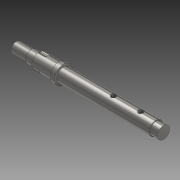
# Autodesk Inventor part: thumb_03 CMC shaft
Saved by Autodesk Inventor 2017 SP1 (Build 210196100, 196)
## iProperties
Created: 2018-02-04
Part Number: thumb_03 CMC shaft
Material: Stainless Steel
Document SubType Name: Modeling
Designer: JT
Density: 8 g/cm^3
Appearance: Semi-Polished
Author: JT
Autodesk Inventor part; units mm, degrees
ref_plane "YZ Plane" through (0, 0, 0) normal (1, 0, 0) x (0, 1, 0)
ref_plane "XZ Plane" through (0, 0, 0) normal (0, 1, 0) x (-1, 0, 0)
sketch "Sketch1" plane through (0, 0, 0) normal (0, 0, 1) x (1, 0, 0)
  line L0 (7.5, 2.5) -> (14, 2.5)
  line L1 (15.5, 2.25) -> (46, 2.25)
  line L2 (46, 2.25) -> (46, 2)
  line L3 (46, 2) -> (48.5, 2)
  line L4 (7.5, 2.5) -> (7.5, 2)
  line L5 (7.5, 2) -> (5, 2)
  line L6 (0, 0) -> (48.5, 0)
  line L7 (48.5, 0) -> (48.5, 2)
  line L8 (14, 2.5) -> (14, 2.95)
  line L9 (14, 2.95) -> (15.5, 2.95)
  line L10 (15.5, 2.95) -> (15.5, 2.25)
  line L11 (5, 2) -> (5, 1.75)
  line L12 (5, 1.75) -> (0, 1.75)
  line L13 (0, 1.75) -> (0, 0)
  dimension "d37" = 3.7
  dimension "d45" = 7.34
  dimension "d4" = 2.5
  dimension "d5" = 4.5
  dimension "d6" = 5
  dimension "d7" = 4
  dimension "d8" = 4
  dimension "d12" = 32
  dimension "d13" = 6.5
  dimension "d14" = 1.5
  dimension "d15" = 5.9
  dimension "d25" = 2.5
  dimension "d26" = 5
  dimension "d27" = 3.5
  constraints: 28 end point, 8 perpendicular, 3 vertical, 1 parallel
  measures "d4" distance between parallel lines of L7 L2
  measures "d5" diameter of L1 L6
  measures "d6" diameter of L0 L6
  measures "d7" diameter of L3 L6
  measures "d8" diameter of L5 L6
  measures "d12" distance between parallel lines of L2 L8
  measures "d13" distance between parallel lines of L8 L4
  measures "d14" distance between parallel lines of L10 L8
  measures "d15" diameter of L9 L6
  measures "d25" distance between parallel lines of L4 L11
  measures "d26" distance between parallel lines of L11 L13
  measures "d27" diameter of L12 L6
revolve "Revolution1" add sketch "Sketch1" angle 360 about axis through (0, 0, 0) along (1, 0, 0)
ref_plane "Work Plane1" through (30.75, 0, -2.25) normal (0, 0, 1) x (1, 0, 0)
sketch "Sketch2" plane through (30.75, 0, -2.25) normal (0, 0, 1) x (1, 0, 0)
  line L0 (-16.75, -2.95) -> (-16.75, 2.95) projected
  line L1 (-30.75, 0) -> (16.721, 0) construction
  point P0 (1.25, 0)
  point P1 (10.25, 0)
  dimension "d16" = 18
  dimension "d17" = 27
  constraints: 2 end point, 2 point on line, 1 horizontal
  measures "d16" distance from line of point (1.25, 0) L0
  measures "d17" distance from line of point (10.25, 0) L0
hole "Hole1" at (32, 0, -2.25) at (41, 0, -2.25) direction (0, 0, 1) diameter 1.6 end through all
sketch "Sketch4" plane through (14, 0, 0) normal (-1, 0, 0) x (0, 0, 1)
  line L0 (0.75, -2.95) -> (-0.75, -2.95)
  line L1 (-0.75, -2.95) -> (-0.75, -10)
  line L2 (-0.75, -10) -> (0.75, -10)
  line L3 (0.75, -10) -> (0.75, -2.95)
  line L4 (0, 0) -> (0, -9.1569) construction
  dimension "d28" = 1.5
  dimension "d29" = 2.95
  dimension "d30" = 10
  constraints: 10 end point, 2 parallel, 1 horizontal, 1 perpendicular, 1 vertical, 1 other
  measures "d28" distance between parallel lines of L1 L3
  measures "d29" distance from line of L4.start L0
  measures "d30" distance from line of L4.start L2
extrude "Extrusion1" [suppressed]
pattern_circular "Circular Pattern1" [suppressed]
sketch "Sketch5" plane through (7.5, 0, 0) normal (-1, 0, 0) x (0, 0, 1)
  line L0 (1.4255, 3.4144) -> (3.6697, 0.4727) construction
  line L1 (3.6697, 0.4727) -> (2.2442, -2.9417) construction
  line L2 (2.2442, -2.9417) -> (-1.4255, -3.4144) construction
  line L3 (-1.4255, -3.4144) -> (-3.6697, -0.4727) construction
  line L4 (-3.6697, -0.4727) -> (-2.2442, 2.9417) construction
  line L5 (-2.2442, 2.9417) -> (1.4255, 3.4144) construction
  line L6 (0, 0) -> (11.1686, 0) construction
  dimension "d37" = 3.7
  dimension "d45" = 7.34
  constraints: 14 end point, 1 coincident, 1 horizontal, 13 other
  measures "d37" distance of L0.start L0.end
  measures "d45" angle of L6 L2
hole "Hole2" at (7.5, -3.4144, -1.4255) at (7.5, 0.4727, 3.6697) at (7.5, 2.9417, -2.2442) direction (1, 0, 0) diameter 3 depth 2.5
sketch "Sketch6" plane through (0, 0, 0) normal (-1, 0, 0) x (0, 0, 1)
  circle A0 centre (0, 0) radius 1.75 projected
  line L0 (-0.75, -1.5811) -> (-0.75, 1.5811)
  dimension "d46" = 0.75
  constraints: 2 end point, 2 point on circle, 1 vertical
  measures "d46" distance from line of point (0, 0) L0
extrude "Extrusion2" cut sketch "Sketch6" against normal up to surface (5 mm away) contours L0 A0 picked at (-1.0833, 0)
body "Solid1"
